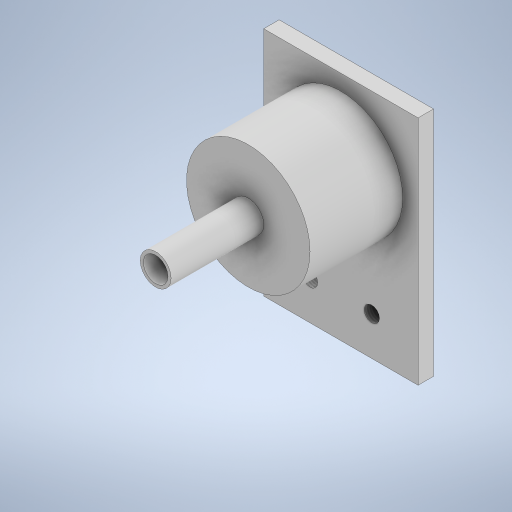
# Autodesk Inventor part: Pump
Saved by Autodesk Inventor 2024 (Build 280153000, 153)
## iProperties
Created: 2024-02-05
Part Number: Pump
Material: Generic
Document SubType Name: Modeling
Designer: Ramji Yadav
Density: 1 g/cm^3
Appearance: Default
Author: Ramji Yadav
Autodesk Inventor part; units mm, degrees
ref_plane "YZ Plane" through (0, 0, 0) normal (1, 0, 0) x (0, 1, 0)
ref_plane "XZ Plane" through (0, 0, 0) normal (0, 1, 0) x (-1, 0, 0)
ref_plane "XY Plane" through (0, 0, 0) normal (0, 0, 1) x (1, 0, 0)
sketch "Sketch1" plane through (0, 0, 0) normal (0, 0, 1) x (1, 0, 0)
  line L0 (0, 0) -> (50, 0)
  line L1 (50, 0) -> (50, 75)
  line L2 (50, 75) -> (0, 75)
  line L3 (0, 75) -> (0, 0)
  dimension "d0" = 50
  dimension "d1" = 75
  constraints: 8 end point, 2 parallel, 1 horizontal, 1 perpendicular
  measures "d0" distance of L2.end L1.end
  measures "d1" distance of L1.end L0.end
extrude "Extrusion1" add sketch "Sketch1" along normal blind 5
sketch "Sketch2" plane through (0, 0, 5) normal (0, 0, 1) x (1, 0, 0)
  line L0 (0, 0) -> (50, 0) projected
  line L1 (50, 75) -> (0, 75) projected
  line L2 (0, 0) -> (50, 0)
  line L3 (50, 0) -> (50, 75)
  line L4 (50, 75) -> (0, 75)
  line L5 (0, 75) -> (0, 0)
  circle A0 centre (25, 50) radius 20
  dimension "d4" = 40
  dimension "d5" = 25
  constraints: 8 end point, 2 parallel, 1 centre point, 1 horizontal, 1 perpendicular
  measures "d4" diameter of A0
  measures "d5" distance from line of L1 A0.centre
extrude "Extrusion2" add sketch "Sketch2" along normal blind 30 contours A0
sketch "Sketch3" plane through (25, 50, 35) normal (0, 0, 1) x (1, 0, 0)
  circle A0 centre (0, 0) radius 4
  circle A1 centre (0, 0) radius 5
  point P0 (-25, -50)
  dimension "d8" = 8
  dimension "d9" = 10
  constraints: 2 centre point, 1 coincident
  measures "d8" diameter of A0
  measures "d9" diameter of A1
extrude "Extrusion3" add sketch "Sketch3" along normal blind 30
sketch "Sketch4" plane through (0, 0, 5) normal (0, 0, 1) x (1, 0, 0)
  circle A0 centre (35, 12.5) radius 2.5
  circle A1 centre (15, 12.5) radius 2.5
  line L0 (0, 75) -> (0, 0) projected
  line L1 (50, 0) -> (50, 75) projected
  line L2 (0, 0) -> (50, 0) projected
  dimension "d12" = 5
  dimension "d13" = 5
  dimension "d14" = 15
  dimension "d15" = 15
  dimension "d16" = 12.5
  dimension "d17" = 12.5
  constraints: 2 centre point
  measures "d12" diameter of A0
  measures "d13" diameter of A1
  measures "d14" distance from line of A1.centre L0
  measures "d15" distance from line of L1 A0.centre
  measures "d16" distance from line of L2 A0.centre
  measures "d17" distance from line of L2 A1.centre
extrude "Extrusion4" cut sketch "Sketch4" against normal blind 10
thread "Thread1" size "M5x0.8" class "6H" standard "ANSI Metric M Profile" full length
thread "Thread2" size "M5x0.8" class "6H" standard "ANSI Metric M Profile" full length
body "Solid1"
